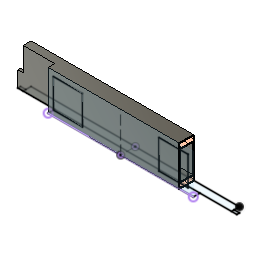
design (Autodesk Fusion 360 design; units mm, degrees)
Autodesk Fusion 360 part; units mm, degrees
sketch "Sketch1" plane through (0, 0, 0) normal (0, 0, 1) x (1, 0, 0) in component "Component'"
  line L0 (-39.5, 0) -> (39.5, 0)
  line L1 (-39.5, 0) -> (-39.5, -2)
  line L2 (-39.5, -2) -> (-41.5, -2)
  line L3 (-41.5, -2) -> (-41.5, -3)
  line L4 (0, 0) -> (0, -5.5) construction
  line L5 (39.5, 0) -> (39.5, -2)
  line L6 (39.5, -2) -> (41.5, -2)
  line L7 (41.5, -2) -> (41.5, -3)
  line L8 (-41.5, -3) -> (41.5, -3)
  line L9 (-27.5, -5.5) -> (27.5, -5.5)
  line L10 (27.5, -5.5) -> (27.5, -3)
  line L11 (-27.5, -5.5) -> (-27.5, -3)
  line L12 (-39.5, -2) -> (-39.5, -3)
  line L13 (39.5, -2) -> (39.5, -3)
  dimension "d19" = 79
  dimension "d20" = 2
  dimension "d21" = 2
  dimension "d22" = 1
  dimension "d23" = 5.5
  dimension "d24" = 55
  constraint horizontal L0
  constraint midpoint L4.start L0
  constraint perpendicular L0 L1
  constraint perpendicular L1 L2
  constraint perpendicular L2 L3
  constraint coincident L4.start origin
  constraint perpendicular L0 L4
  constraint symmetric L0.start L4 L0.end
  constraint symmetric L1.end L4 L5.end
  constraint symmetric L2.end L4 L6.end
  constraint symmetric L3.end L4 L7.end
  constraint horizontal L9
  constraint midpoint L4.end L9
  constraint coincident L8 L10.end
  constraint perpendicular L8 L10
  constraint coincident L8 L11.end
  constraint perpendicular L8 L11
  constraint coincident L8 L12.end
  constraint perpendicular L8 L12
  constraint coincident L8 L13.end
  constraint perpendicular L8 L13
  measures "d19" distance of L0.start L0.end
  measures "d20" distance of L0.start L1.end
  measures "d21" distance of L1.end L2.end
  measures "d22" distance of L2.end L3.end
  measures "d23" distance of L4.start L4.end
  measures "d24" distance of L9.start L9.end
extrude "Extrude1" add sketch "Sketch1" along normal blind 15 contours L0 L1 L5 L8 L12 L13 | L8 L9 L10 L11 in component "Component'"
extrude "Extrude2" add sketch "Sketch1" along normal blind 6 contours L2 L3 L8 L12 | L6 L7 L8 L13 in component "Component'"
sketch "Sketch2" plane through (0, -5.5, 0) normal (0, -1, 0) x (1, 0, 0) in component "Component'"
  line L0 (-27.5, 0) -> (27.5, 0)
  line L1 (27.5, 0) -> (27.5, 15)
  line L2 (27.5, 15) -> (-27.5, 15)
  line L3 (-27.5, 15) -> (-27.5, 0)
  line L4 (-25.5, 13) -> (-14.5, 13)
  line L5 (-14.5, 13) -> (-14.5, 2)
  line L6 (-14.5, 2) -> (-25.5, 2)
  line L7 (-25.5, 2) -> (-25.5, 13)
  line L8 (-27.5, 0) -> (27.5, 0)
  line L9 (0, 0) -> (0, 15) construction
  line L10 (25.5, 13) -> (14.5, 13)
  line L11 (25.5, 2) -> (25.5, 13)
  line L12 (14.5, 13) -> (14.5, 2)
  line L13 (14.5, 2) -> (25.5, 2)
  dimension "d29" = 11
  dimension "d30" = 11
  dimension "d31" = 2
  dimension "d32" = 2
  constraint horizontal L4
  constraint vertical L5
  constraint horizontal L6
  constraint vertical L7
  constraint coincident L9.start origin
  constraint midpoint L2 L9.end
  constraint symmetric L4.start L9 L10.start
  constraint symmetric L4.end L9 L10.end
  constraint symmetric L5.end L9 L12.end
  constraint symmetric L6.end L9 L11.start
  measures "d29" distance of L4.start L4.end
  measures "d30" distance of L4.start L6.end
  measures "d31" distance of L3 L7
  measures "d32" distance of L6 L8
extrude "Extrude3" cut sketch "Sketch2" against normal up to surface (5.5 mm away) contours L4 L5 L6 L7 | L10 L11 L12 L13 in component "Component'"
sketch "Sketch3" plane through (0, 0, 15) normal (0, 0, 1) x (-1, 0, 0) in component "Component'"
  line L0 (39.5, 0) -> (39.5, 3)
  line L1 (39.5, 3) -> (27.5, 3)
  line L2 (27.5, 3) -> (27.5, 5.5)
  line L3 (27.5, 5.5) -> (-27.5, 5.5)
  line L4 (-27.5, 5.5) -> (-27.5, 3)
  line L5 (-27.5, 3) -> (-39.5, 3)
  line L6 (-39.5, 3) -> (-39.5, 0)
  line L7 (-39.5, 0) -> (39.5, 0)
  line L8 (39.5, 0.3) -> (-39.5, 0.3)
  line L9 (27.5, 5.2) -> (-27.5, 5.2)
  line L10 (39.5, 0) -> (-39.5, 0)
  line L11 (27.5, 5.5) -> (-27.5, 5.5)
  dimension "d36" = 0.3
  dimension "d37" = 0.3
  constraint coincident L0 L8.start
  constraint coincident L6 L8.end
  constraint perpendicular L6 L8
  constraint coincident L2 L9.start
  constraint coincident L4 L9.end
  constraint perpendicular L4 L9
  measures "d36" distance of L8 L10
  measures "d37" distance of L9 L11
extrude "Extrude4" add sketch "Sketch3" against normal up to surface (15 mm away) contours L0 L6 L7 L8 L10 | L2 L3 L4 L9 L11 in component "Component'"
component "Component'" placed x (1, 0, 0) y (0, 1, 0) z (0, 0, 1) at (0, 0, 0)
